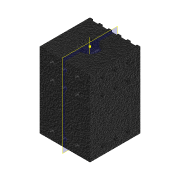
# Autodesk Inventor part: 00_LASER_640nm
Saved by Autodesk Inventor 2022 (Build 260153000, 153)
## iProperties
Created: 2017-07-07
Part Number: 00_LASER_640nm
Material: Generisch
Document SubType Name: Modeling
Designer: diederichbenedict
Density: 1 g/cm^3
Appearance: Schwarz - Guss
Author: diederichbenedict
Autodesk Inventor part; units mm, degrees
ref_plane "YZ Plane" through (0, 0, 0) normal (1, 0, 0) x (0, 1, 0)
ref_plane "XZ Plane" through (0, 0, 0) normal (0, 1, 0) x (-1, 0, 0)
ref_plane "XY Plane" through (0, 0, 0) normal (0, 0, 1) x (1, 0, 0)
sketch "Skizze1" plane through (0, 0, 0) normal (0, 0, 1) x (1, 0, 0)
  line L0 (-16, 16) -> (16, 16)
  line L1 (16, 16) -> (16, -16)
  line L2 (16, -16) -> (-16, -16)
  line L3 (-16, -16) -> (-16, 16)
  line L4 (-16, 16) -> (16, -16) construction
  line L5 (16, 16) -> (-16, -16) construction
  point P0 (0, 0)
  dimension "d0" = 32
  dimension "d1" = 32
  constraints: 12 end point, 2 midpoint, 2 parallel, 1 horizontal, 1 perpendicular
  measures "d0" distance of L1.end L2.end
  measures "d1" distance of L0.end L1.end
extrude "Extrusion1" add sketch "Skizze1" along normal blind 48
sketch "Skizze2" plane through (-16, 16, 0) normal (0, 1, 0) x (1, 0, 0)
  line L0 (0, 0) -> (32, 0) construction
  line L1 (0, 0) -> (0, -48) construction
  line L2 (32, -48) -> (0, -48) construction
  line L3 (32, 0) -> (32, -48) construction
  line L4 (5, -43) -> (5, -5)
  line L5 (5, -5) -> (27, -5)
  line L6 (27, -5) -> (27, -43)
  line L7 (27, -43) -> (5, -43)
  line L8 (32, -48) -> (0, -48) projected
  line L9 (16, -48) -> (16, 0)
  circle A0 centre (16, -5) radius 1.4
  circle A1 centre (24, -5) radius 1.4
  circle A2 centre (16, -43) radius 1.4
  circle A3 centre (8, -43) radius 1.4
  circle A4 centre (24, -43) radius 1.4
  line L10 (27, -33) -> (5, -33)
  circle A5 centre (24, -33) radius 1.4
  circle A6 centre (16, -33) radius 1.4
  circle A7 centre (8, -33) radius 1.4
  circle A8 centre (8, -5) radius 1.4
  dimension "d4" = 5
  dimension "d5" = 2.8
  dimension "a1" = 2.8
  dimension "d8" = 2.8
  dimension "d10" = 8
  dimension "d11" = 2.8
  dimension "d12" = 2.8
  dimension "d23" = 10
  dimension "d40" = 8
  dimension "d41" = 8
  dimension "d42" = 8
  dimension "d43" = 8
  dimension "d44" = 2.8
  dimension "d45" = 2.8
  dimension "d46" = 2.8
  dimension "d47" = 2.8
  constraints: 12 end point, 10 point on line, 9 centre point, 4 midpoint, 1 perpendicular, 1 vertical, 3 other
  measures "d4" distance between parallel lines of L1 L4
  measures "d5" diameter of A0
  measures "a1" diameter of A1
  measures "d8" diameter of A2
  measures "d10" distance of A1.centre A0.centre
  measures "d11" diameter of A3
  measures "d12" diameter of A4
  measures "d23" distance between parallel lines of L10 L7
  measures "d40" distance of A2.centre A3.centre
  measures "d41" distance of A4.centre A2.centre
  measures "d42" distance of A5.centre A6.centre
  measures "d43" distance of A6.centre A7.centre
  measures "d44" diameter of A8
  measures "d45" diameter of A7
  measures "d46" diameter of A6
  measures "d47" diameter of A5
extrude "Extrusion2" cut sketch "Skizze2" against normal through all contours A3 L7 | L7 A3 | A7 L10 | L10 A7 | A8 L5 | L5 A8 | A2 L9 L7 | L7 L9 A2 | A6 L9 L10 | L10 L9 A6 | L9 A2 L7 | L7 A2 L9 | A0 L9 L5 | L5 L9 A0 | L10 A6 L9 | L9 A6 L10 | L9 A0 L5 | L5 A0 L9 | A4 L7 | L7 A4 | A5 L10 | L10 A5 | A1 L5 | L5 A1
sketch "Skizze3" plane through (0, 0, 48) normal (0, 0, 1) x (1, 0, 0)
  circle A0 centre (0, 0) radius 2.5
  dimension "d15" = 5
  constraints: 1 centre point, 1 coincident
  measures "d15" diameter of A0
extrude "Extrusion3" cut sketch "Skizze3" against normal through all
sketch "Skizze4" plane through (0, 0, 48) normal (0, 0, 1) x (1, 0, 0)
  line L0 (-2.45, 0.55) -> (-42.45, 0.55) projected
  circle A0 centre (0, 0) radius 2.5 projected
  line L1 (16, 16) -> (-16, 16) projected
  line L2 (-16, 16) -> (-16, -16) projected
  line L3 (-16, -16) -> (16, -16) projected
  line L4 (16, -16) -> (16, 16) projected
  circle A1 centre (0, 0) radius 6
  dimension "d18" = 12
  constraints: 1 centre point, 1 coincident
  measures "d18" diameter of A1
extrude "Extrusion4" cut sketch "Skizze4" against normal blind 5 contours A1
pattern_circular "Runde Anordnung1" count 4 over 360 about axis through (0, 0, 48) along (0, 0, -1) of "Extrusion2"
sketch "Sketch6" plane through (0, 0, 48) normal (0, 0, 1) x (1, 0, 0)
  point P0 (0, 0)
sketch "Sketch7" plane through (-16, 16, 0) normal (0, 1, 0) x (1, 0, 0)
  circle A0 centre (8, -33) radius 1.4 projected
  circle A1 centre (16, -33) radius 1.4 projected
  circle A2 centre (24, -43) radius 1.4 projected
  circle A3 centre (16, -43) radius 1.4 projected
  circle A4 centre (16, -5) radius 1.4 projected
  circle A5 centre (24, -5) radius 1.4 projected
  circle A6 centre (8, -43) radius 1.4 projected
  circle A7 centre (24, -33) radius 1.4 projected
  circle A8 centre (8, -5) radius 1.4 projected
  line L0 (0, 0) -> (32, 0) projected
  line L1 (0, 0) -> (0, -48) projected
  line L2 (32, -48) -> (0, -48) projected
  line L3 (32, 0) -> (32, -48) projected
  line L4 (22, -48) -> (10, -48) projected
  line L5 (18, 0) -> (14, 0)
  line L6 (14, 0) -> (14, -48)
  line L7 (14, -48) -> (18, -48)
  line L8 (18, -48) -> (18, 0)
  point P0 (16, 0)
  dimension "d48" = 2
  dimension "d49" = 2
  constraints: 8 end point, 2 parallel, 2 point on line, 1 horizontal, 1 perpendicular
  measures "d48" distance from line of A4.centre L8
  measures "d49" distance from line of L6 A4.centre
extrude "Extrusion6" cut sketch "Sketch7" against normal blind 1 contours L0 L8 L2 L6
pattern_linear "Rectangular Pattern1" count 3 spacing 6 along (-1, 0, 0) count 3 spacing 6 along (1, 0, 0) of "Extrusion6"
ref_plane "Work Plane1" through (0, -16, 0) normal (-1, 0, 0) x (0, 0, 1)
ref_plane "Work Plane2" through (0, 0, 24) normal (0, 0, -1) x (-1, 0, 0)
equation "\"d5\" = a1"
equation "\"d8\" = a1"
equation "\"d11\" = a1"
equation "\"d12\" = a1"
equation "\"d44\" = a1"
equation "\"d45\" = a1"
equation "\"d46\" = a1"
equation "\"d47\" = a1"
